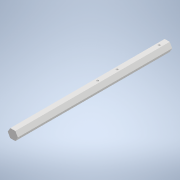
# Autodesk Inventor part: Eje_Entrada
Saved by Autodesk Inventor 2022 (Build 260153000, 153)
## iProperties
Created: 2022-02-21
Part Number: Eje_Entrada
Material: Generic
Document SubType Name: Modeling
Designer: katha
Density: 1 g/cm^3
Appearance: Default
Author: katha
Autodesk Inventor part; units mm, degrees
ref_plane "YZ Plane" through (0, 0, 0) normal (1, 0, 0) x (0, 1, 0)
ref_plane "XZ Plane" through (0, 0, 0) normal (0, 1, 0) x (-1, 0, 0)
ref_plane "XY Plane" through (0, 0, 0) normal (0, 0, 1) x (1, 0, 0)
sketch "Sketch7" plane through (0, 0, 0) normal (0, 0, 1) x (1, 0, 0)
  line L0 (0, 0) -> (3.1, 0) construction
  circle A0 centre (0, 0) radius 3.1 construction
  line L1 (0, 0) -> (1.55, 2.6847) construction
  line L2 (0, 0) -> (-1.55, 2.6847) construction
  line L3 (0, 0) -> (-3.1, 0) construction
  line L4 (0, 0) -> (-1.55, -2.6847) construction
  line L5 (0, 0) -> (1.55, -2.6847) construction
  line L6 (-1.55, 2.6847) -> (1.55, 2.6847)
  line L7 (1.55, 2.6847) -> (3.1, 0)
  line L8 (3.1, 0) -> (1.55, -2.6847)
  line L9 (1.55, -2.6847) -> (-1.55, -2.6847)
  line L10 (-1.55, -2.6847) -> (-3.1, 0)
  line L11 (-3.1, 0) -> (-1.55, 2.6847)
  dimension "d17" = 3.1
  dimension "d20" = 360
  constraints: 24 end point, 3 parallel, 2 horizontal, 2 point on circle, 1 centre point, 1 coincident, 19 other
  measures "d17" distance of L0.start L0.end
extrude "Extrusion5" add sketch "Sketch7" along normal blind 95
sketch "Sketch8" plane through (-1.55, 2.6847, 0) normal (0, 1, 0) x (1, 0, 0)
  line L0 (3.1, -95) -> (0, -95) construction
  line L1 (3.1, 0) -> (0, 0) construction
  line L2 (0, -95) -> (3.1, -95) projected
  line L3 (1.55, -95) -> (1.55, 0) construction
  circle A0 centre (1.55, -30.9) radius 0.65
  circle A1 centre (1.55, -42.9) radius 0.65
  circle A2 centre (1.55, -5) radius 0.65
  dimension "d24" = 1.3
  dimension "d25" = 64.1
  dimension "d26" = 52.1
  dimension "d29" = 5
  constraints: 3 centre point, 3 point on line, 2 end point, 2 equal radius, 1 midpoint, 1 perpendicular
  measures "d24" diameter of A0
  measures "d25" distance of A0.centre L3.start
  measures "d26" distance of A1.centre L3.start
  measures "d29" distance from line of L1 A2.centre
extrude "Extrusion6" cut sketch "Sketch8" against normal blind 6
body "Solid2"
